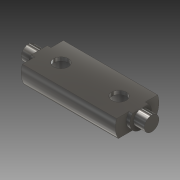
# Autodesk Inventor part: 0th_finger_mount
Saved by Autodesk Inventor 2017 SP1 (Build 210196100, 196)
## iProperties
Created: 2017-06-21
Part Number: 0th_finger_mount
Material: Generic
Document SubType Name: Modeling
Designer: Tomasz
Density: 1 g/cm^3
Appearance: Steel - Polished
finger_mounting_screw_distance: 8,000 mm
finger_shaft_diameter: 6,000 mm
finger_inner_width: 14,000 mm
Author: Tomasz
Autodesk Inventor part; units mm, degrees
ref_plane "YZ Plane" through (0, 0, 0) normal (1, 0, 0) x (0, 1, 0)
ref_plane "XZ Plane" through (0, 0, 0) normal (0, 1, 0) x (-1, 0, 0)
sketch "Sketch1" plane through (0, 0, 0) normal (0, 0, 1) x (1, 0, 0)
  line L0 (0, 0) -> (8.5, 0)
  line L1 (0, 0) -> (0, 1)
  line L2 (0, 1) -> (1.5, 1)
  line L3 (1.5, 1) -> (1.5, 1.5)
  line L4 (1.5, 1.5) -> (2, 1.5)
  line L5 (2, 1.5) -> (2, 3)
  line L6 (8.5, 0) -> (8.5, 8.9525) construction
  line L7 (2, 3) -> (8.5, 3)
  line L8 (17, 0) -> (8.5, 0)
  line L9 (17, 0) -> (17, 1)
  line L10 (17, 1) -> (15.5, 1)
  line L11 (15.5, 1) -> (15.5, 1.5)
  line L12 (15.5, 1.5) -> (15, 1.5)
  line L13 (15, 1.5) -> (15, 3)
  line L14 (15, 3) -> (8.5, 3)
  dimension "d0" = 7
  dimension "d1" = 1
  dimension "d2" = 1.5
  dimension "d3" = 1.5
  dimension "d4" = 3
  dimension "d5" = 0.5
  constraints: 32 end point, 6 symmetric about line, 5 perpendicular, 2 vertical, 1 horizontal, 1 point on line
  measures "d0" distance from line of L6 L3.end
  measures "d1" distance between parallel lines of L0 L2
  measures "d2" distance between parallel lines of L4 L0
  measures "d3" distance from line of L2.end L1
  measures "d4" distance between parallel lines of L7 L0
  measures "d5" distance between parallel lines of L5 L3
revolve "Revolution1" add sketch "Sketch1" angle 360 about axis through (0, 0, 0) along (1, 0, 0)
ref_plane "Work Plane1" through (0.75, 0, 1) normal (0, 0, 1) x (1, 0, 0)
sketch "Sketch2" plane through (0.75, 0, 1) normal (0, 0, 1) x (1, 0, 0)
  line L0 (1.25, -3) -> (1.25, 3) projected
  line L1 (14.25, -3) -> (14.25, 3) projected
  line L2 (0.75, -1.5) -> (0.75, 1.5) projected
  line L3 (1.25, -1.5) -> (1.25, 1.5) projected
  line L4 (14.25, -1.5) -> (14.25, 1.5) projected
  line L5 (14.75, -1.5) -> (14.75, 1.5) projected
  line L6 (0.75, 1.5) -> (1.25, 1.5) projected
  line L7 (0.75, -1.5) -> (1.25, -1.5) projected
  line L8 (14.25, 1.5) -> (14.75, 1.5) projected
  line L9 (14.25, -1.5) -> (14.75, -1.5) projected
  line L10 (1.25, -3) -> (14.25, -3) projected
  line L11 (1.25, 3) -> (14.25, 3) projected
  point P0 (-0.75, 0)
extrude "Extrusion1" cut sketch "Sketch2" along normal through all
ref_plane "Work Plane2" through (1.75, 0, -1.5) normal (0, 0, 1) x (1, 0, 0)
sketch "Sketch3" plane through (1.75, 0, -1.5) normal (0, 0, 1) x (1, 0, 0)
  line L0 (0.25, 3) -> (13.25, 3) projected
  line L1 (13.25, -3) -> (13.25, 3) projected
  line L2 (0.25, -3) -> (0.25, 3) projected
  line L3 (0.25, -3) -> (13.25, -3) projected
  point P0 (-1.75, 0)
  point P1 (13.25, -2.8284)
  point P2 (13.25, 2.8284)
  point P3 (0.25, -2.8284)
  point P4 (0.25, 2.8284)
extrude "Extrusion2" cut sketch "Sketch3" against normal through all
sketch "Sketch4" plane through (1.75, 0, -1.5) normal (0, 0, 1) x (1, 0, 0)
  line L0 (15.25, -1) -> (15.25, 1) projected
  line L1 (15.25, 0) -> (-1.75, 0) construction
  line L2 (6.75, 0) -> (6.75, 2.8511) construction
  line L3 (-1.75, 0) -> (15.25, 0) construction
  point P0 (10.75, 0)
  point P1 (2.75, 0)
  dimension "d11" = 8
  constraints: 6 end point, 3 symmetric about line, 2 midpoint, 2 point on line, 1 horizontal, 1 vertical
  measures "d11" distance of point (2.75, 0) point (10.75, 0)
hole "Hole1" at (12.5, 0, -1.5) at (4.5, 0, -1.5) direction (0, 0, 1) diameter 2 end through all counterbore diameter 4 counterbore depth 2
equation "\"d0\" = 0.5 * finger_inner_width"
equation "\"d4\" = 0.5 * finger_shaft_diameter"
equation "\"d11\" = finger_mounting_screw_distance"
equation "\"finger_mounting_screw_distance\" = 8"
equation "\"finger_shaft_diameter\" = 6"
equation "\"finger_inner_width\" = 14"
body "Solid1"
